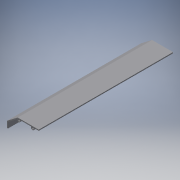
# Autodesk Inventor part: DriveBaseFront
Saved by Autodesk Inventor 2017 (Build 210142000, 142)
## iProperties
Created: 2017-04-25
Part Number: DriveBaseFront
Material: Generic
Document SubType Name: Modeling
Designer: admin
Density: 1 g/cm^3
Appearance: Default
Author: admin
Autodesk Inventor part; units mm, degrees
ref_plane "YZ Plane" through (0, 0, 0) normal (1, 0, 0) x (0, 1, 0)
ref_plane "XZ Plane" through (0, 0, 0) normal (0, 1, 0) x (-1, 0, 0)
ref_plane "XY Plane" through (0, 0, 0) normal (0, 0, 1) x (1, 0, 0)
ref_plane "Work Plane1" through (0, 0, 0) normal (0, 0, 1) x (1, 0, 0)
sketch "Sketch1" plane through (0, 0, 0) normal (0, 0, 1) x (1, 0, 0)
  line L0 (41.7899, 406.4) -> (106.8774, 406.4) projected
  line L1 (14.8024, 385.8381) -> (41.7899, 406.4) projected
  line L2 (106.8774, 403.225) -> (42.8616, 403.225)
  line L3 (42.8616, 403.225) -> (16.7266, 383.3126)
  line L4 (106.8774, 406.4) -> (106.8774, 403.225)
  line L5 (11.6274, 361.95) -> (11.6274, 80.1687) projected
  line L6 (16.7266, 383.3126) -> (11.6274, 379.4275)
  line L7 (14.8024, 385.8381) -> (8.4524, 381)
  line L8 (11.6274, 361.95) -> (11.6274, 379.4275)
  line L9 (11.6274, 361.95) -> (11.6274, 80.1687) projected
  line L10 (8.4524, 361.95) -> (8.4524, 80.1687) projected
  line L11 (11.6274, 361.95) -> (8.4524, 361.95) projected
  line L12 (8.4524, 361.95) -> (8.4524, 381)
  point P0 (0, 0)
  dimension "d0" = 3.175
  constraints: 14 end point, 3 vertical, 1 collinear, 1 other
  measures "d0" distance between parallel lines of L0 L2
extrude "Extrusion1" add sketch "Sketch1" along normal blind 415.925
sketch "Sketch2" plane through (0, 0, 415.925) normal (0, 0, 1) x (1, 0, 0)
  line L0 (42.8616, 403.225) -> (106.8774, 403.225) projected
  line L1 (92.9074, 403.225) -> (82.7474, 403.225)
  arc A0 (82.7474, 400.685) -> (92.9074, 400.685) centre (87.8274, 400.685) ccw
  line L2 (106.8774, 406.4) -> (41.7899, 406.4) projected
  arc A1 (89.5122, 403.225) -> (86.1425, 403.225) centre (87.8274, 400.685) ccw
  line L3 (92.9074, 400.685) -> (92.9074, 403.225)
  line L4 (82.7474, 403.225) -> (82.7474, 400.685)
  arc A2 (83.428, 403.225) -> (82.7474, 400.685) centre (87.8274, 400.685) ccw construction
  arc A3 (92.2268, 403.225) -> (83.428, 403.225) centre (87.8274, 400.685) ccw
  arc A4 (92.9074, 400.685) -> (92.2268, 403.225) centre (87.8274, 400.685) ccw construction
  arc A5 (86.1425, 403.225) -> (89.5122, 403.225) centre (87.8274, 400.685) ccw
  line L5 (41.1835, 405.938) -> (43.2506, 403.225)
  line L6 (14.8024, 385.8381) -> (41.7899, 406.4) projected
  arc A6 (40.1058, 400.685) -> (50.2658, 400.685) centre (45.1858, 400.685) ccw
  arc A7 (43.501, 403.225) -> (46.8707, 403.225) centre (45.1858, 400.685) ccw
  line L7 (50.2658, 400.685) -> (50.2658, 403.225)
  line L8 (11.6274, 379.4275) -> (42.8616, 403.225) projected
  line L9 (40.1058, 400.685) -> (40.1058, 401.1254)
  line L10 (43.2506, 403.225) -> (43.3386, 403.1095) construction
  arc A8 (40.1264, 401.141) -> (40.1058, 400.685) centre (45.1858, 400.685) ccw construction
  arc A9 (49.5853, 403.225) -> (40.1264, 401.141) centre (45.1858, 400.685) ccw
  arc A10 (50.2658, 400.685) -> (49.5853, 403.225) centre (45.1858, 400.685) ccw construction
  arc A11 (46.8707, 403.225) -> (43.501, 403.225) centre (45.1858, 400.685) ccw
  point P0 (0, 0)
  dimension "d3" = 10.16
  dimension "d4" = 13.97
  dimension "d5" = 10.16
  dimension "d8" = 6.096
  dimension "d9" = 5.715
  dimension "d10" = 3.556
  dimension "d11" = 10.16
  dimension "d12" = 6.096
  dimension "d13" = 5.715
  constraints: 27 point on circle, 14 end point, 12 centre point, 12 tangent, 7 point on line, 3 vertical, 2 coincident, 2 line through centre, 2 perpendicular, 8 other
  measures "d3" distance of L1.start L1.end
  measures "d4" distance of L1.start point (106.877, 403.225)
  measures "d5" diameter of A0
  measures "d8" diameter of A1
  measures "d9" distance from line of L2 A1.centre
  measures "d10" distance of L5.start L10.end
  measures "d11" diameter of A6
  measures "d12" diameter of A7
  measures "d13" distance from line of L2 A6.centre
extrude "Extrusion2" add sketch "Sketch2" against normal up to surface (415.925 mm away) contours L0 A7 L7 A6 L9 L8 | L0 A5 L3 A0 L4
body "Solid1"
